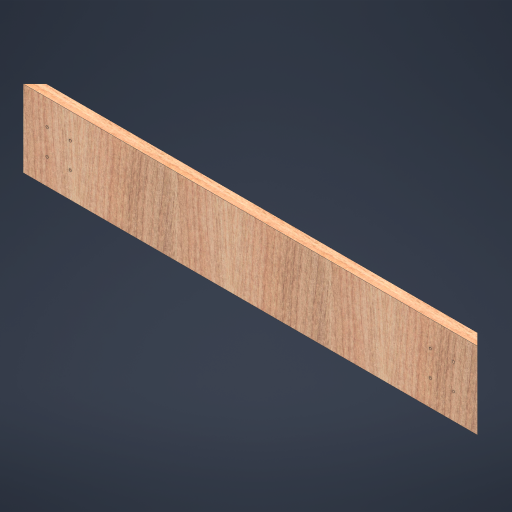
# Autodesk Inventor part: BUMP_001_Wood1
Saved by Autodesk Inventor 2024.2 (Build 282272000, 272)
## iProperties
Created: 2024-08-06
Part Number: BUMP_001_Wood1
Material: Wood (Birch)
Document SubType Name: Modeling
Designer: Bryan
Density: 0.55 g/cm^3
Appearance: Birch - Natural Polished
Author: Bryan
Autodesk Inventor part; units mm, degrees
ref_plane "YZ Plane" through (0, 0, 0) normal (1, 0, 0) x (0, 1, 0)
ref_plane "XZ Plane" through (0, 0, 0) normal (0, 1, 0) x (-1, 0, 0)
ref_plane "XY Plane" through (0, 0, 0) normal (0, 0, 1) x (1, 0, 0)
sketch "Sketch1" plane through (0, 0, 0) normal (0, 1, 0) x (-1, 0, 0)
  line L0 (-355.6, -406.4) -> (355.6, -406.4) construction
  line L1 (355.6, -406.4) -> (355.6, 406.4) construction
  line L2 (355.6, 406.4) -> (-355.6, 406.4)
  line L3 (-355.6, 406.4) -> (-355.6, -406.4) construction
  line L4 (-355.6, -406.4) -> (355.6, 406.4) construction
  line L5 (355.6, -406.4) -> (-355.6, 406.4) construction
  line L6 (374.65, 425.45) -> (374.65, -425.45) construction
  line L7 (374.65, -425.45) -> (-374.65, -425.45) construction
  line L8 (-374.65, -425.45) -> (-374.65, 425.45) construction
  line L9 (-374.65, 425.45) -> (374.65, 425.45)
  line L10 (374.65, 425.45) -> (355.6, 406.4)
  line L11 (-355.6, 406.4) -> (-374.65, 425.45)
  point P0 (0, 0)
  dimension "d0" = 711.2
  dimension "d1" = 812.8
  dimension "d2" = 19.05
  constraints: 24 end point, 4 parallel, 2 midpoint, 2 perpendicular, 1 horizontal, 3 other
  measures "d0" distance of L2.end L1.end
  measures "d1" distance of L1.end L0.end
  measures "d2" distance between parallel lines of L1 L6
extrude "Extrusion1" add sketch "Sketch1" along normal blind 127
sketch "Sketch2" plane through (355.6, 0, 406.4) normal (0, 0, -1) x (-1, 0, 0)
  line L0 (0, 0) -> (711.2, 0) projected
  line L1 (711.2, 0) -> (711.2, 127) projected
  line L2 (0, 127) -> (711.2, 127) projected
  line L3 (0, 0) -> (0, 127) projected
  line L4 (0, 0) -> (0, 127) projected
  circle A0 centre (20.574, 84.6667) radius 1.905
  line L5 (0, 84.6667) -> (20.574, 84.6667) construction
  circle A1 centre (58.674, 84.6667) radius 1.905
  circle A2 centre (96.774, 84.6667) radius 1.905 construction
  circle A3 centre (20.574, 42.3333) radius 1.905
  circle A4 centre (58.674, 42.3333) radius 1.905
  circle A5 centre (96.774, 42.3333) radius 1.905 construction
  line L6 (355.6, 127) -> (355.6, 0) construction
  circle A6 centre (690.626, 84.6667) radius 1.905
  circle A7 centre (652.526, 84.6667) radius 1.905
  circle A8 centre (614.426, 84.6667) radius 1.905 construction
  circle A9 centre (690.626, 42.3333) radius 1.905
  circle A10 centre (652.526, 42.3333) radius 1.905
  circle A11 centre (614.426, 42.3333) radius 1.905 construction
  point P0 (0, 63.5)
  point P1 (0, 63.5)
  dimension "d9" = 3.81
  dimension "d10" = 20.574
  dimension "d11" = 127
  dimension "d12" = 42.3333
  dimension "d16" = 38.1
  dimension "d19" = 42.3333
  constraints: 12 centre point, 7 symmetric about line, 4 end point, 3 midpoint, 2 coincident, 2 horizontal, 2 vertical, 1 point on line, 16 other
  measures "d9" diameter of A0
  measures "d10" distance from line of A0.centre L3
  measures "d11" distance of L0.start L2.start
  measures "d12" distance between parallel lines of L5 L2
  measures "d16" distance of A0.centre A1.centre
  measures "d19" distance of A0.centre A3.centre
extrude "Extrusion2" cut sketch "Sketch2" against normal blind 127 contours A0 | A1 | A3 | A4 | A6 | A7 | A9 | A10
equation "\"d12\" = 0.333333 * d11"
body "Solid1"
